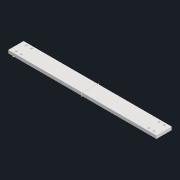
# Autodesk Inventor part: LaminaSoporteAccionadorF
Saved by Autodesk Inventor 2021 (Build 250183000, 183)
## iProperties
Created: 2021-06-15
Part Number: LaminaSoporteAccionadorF
Material: Generic
Document SubType Name: Sheet Metal
Designer: GABRIEL LOL
Density: 1 g/cm^3
Appearance: Default
Sheet Metal Rule: Default
Author: GABRIEL LOL
Autodesk Inventor part; units mm, degrees
ref_plane "YZ Plane" through (0, 0, 0) normal (1, 0, 0) x (0, 1, 0)
ref_plane "XZ Plane" through (0, 0, 0) normal (0, 1, 0) x (-1, 0, 0)
ref_plane "XY Plane" through (0, 0, 0) normal (0, 0, 1) x (1, 0, 0)
sketch "Sketch3" plane through (0, 0, 0) normal (0, 1, 0) x (-1, 0, 0)
  line L0 (5, 0) -> (-140, 0)
  line L1 (-140, 0) -> (-140, -15)
  line L2 (-140, -15) -> (5, -15)
  line L3 (5, -15) -> (5, 0)
  dimension "d6" = 145
  dimension "d7" = 15
  measures "d6" distance of L2.end L1.end
  measures "d7" distance of L1.end L0.end
extrude "Plate1" add sketch "Sketch3" along normal blind 3
sketch "Sketch5" plane through (0, 0, 0) normal (0, -1, 0) x (1, 0, 0)
  line L0 (-5, 0) -> (140, 0) projected
  line L1 (-5, -15) -> (-5, 0) projected
  line L2 (140, -15) -> (-5, -15) projected
  line L3 (140, 0) -> (140, -15) projected
  line L4 (140, 0) -> (140, -15) construction
  line L5 (140, -7.5) -> (135, -7.5) construction
  line L6 (135, -7.5) -> (135, -12.5) construction
  line L7 (135, -12.5) -> (135, -2.5) construction
  line L8 (135, -2.5) -> (130, -2.5) construction
  line L9 (130, -2.5) -> (130, -12.5) construction
  circle A0 centre (135, -2.5) radius 1
  circle A1 centre (135, -12.5) radius 1
  circle A2 centre (130, -2.5) radius 1
  circle A3 centre (130, -12.5) radius 1
  point P0 (0, 0)
  dimension "d19" = 5
  dimension "d20" = 5
  dimension "d21" = 10
  dimension "d22" = 5
  dimension "d23" = 2
  dimension "d24" = 2
  dimension "d25" = 2
  dimension "d26" = 2
  constraints: 10 end point, 4 centre point, 4 coincident, 3 perpendicular, 1 horizontal, 1 midpoint, 1 point on line
  measures "d19" distance of L5.start L5.end
  measures "d20" distance of L5.end L6.end
  measures "d21" distance of L6.end L7.end
  measures "d22" distance of L7.end L8.end
  measures "d23" diameter of A0
  measures "d24" diameter of A1
  measures "d25" diameter of A2
  measures "d26" diameter of A3
extrude "Extrusion2" cut sketch "Sketch5" against normal blind 10 contours A0 | A1 | A2 | A3
sketch "Sketch6" plane through (0, 0, 0) normal (0, -1, 0) x (1, 0, 0)
  point P0 (0, 0)
ref_plane "Work Plane1" through (67.5, 0, 0) normal (1, 0, 0) x (0, 0, -1)
mirror "Mirror1" about plane through (67.5, 0, 0) normal (1, 0, 0) of "Extrusion2"
equation "\"d8\" = Thickness"
equation "\"BendRadius\" = Thickness"
equation "\"BendReliefWidth\" = Thickness"
equation "\"BendReliefDepth\" = 0.5 * Thickness"
equation "\"CornerReliefSize\" = 4 * Thickness"
equation "\"MinimumRemnant\" = 2 * Thickness"
equation "\"TransitionRadius\" = BendRadius"
equation "\"JacobiRadiusSize\" = Thickness"
equation "\"GapSize\" = Thickness"
equation "\"Thickness\" = 3"
body "Solid2"
